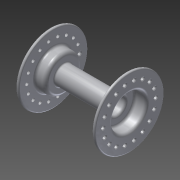
# Autodesk Inventor part: Korpus_piasty
Saved by Autodesk Inventor 2015 (Build 190159000, 159)
## iProperties
Created: 2015-11-24
Part Number: Korpus_piasty
Material: Aluminium AW-7020
Document SubType Name: Modeling
Designer: graaapsik
Density: 2.78 g/cm^3
Appearance: Aluminium AW-7020
Mass: 39.303 g
Surface Area: 181.03 cm^2
Volume: 14.1378 cm^3
Author: graaapsik
Autodesk Inventor part; units mm, degrees
ref_plane "YZ Plane" through (0, 0, 0) normal (1, 0, 0) x (0, 1, 0)
ref_plane "XZ Plane" through (0, 0, 0) normal (0, 1, 0) x (-1, 0, 0)
ref_plane "XY Plane" through (0, 0, 0) normal (0, 0, 1) x (1, 0, 0)
sketch "Szkic1" plane through (0, 0, 0) normal (0, 0, 1) x (1, 0, 0)
  line L0 (-11.9267, 0) -> (11.9804, 0) construction
  line L1 (-21.5, 8) -> (21.5, 8)
  line L2 (0, 16.2765) -> (0, -12.1999) construction
  arc A0 (21.5, 8) -> (22.5, 9) centre (21.5, 9) ccw
  line L3 (22.5, 9) -> (22.5, 12.5)
  arc A1 (25.5, 15.5) -> (22.5, 12.5) centre (25.5, 12.5) ccw
  line L4 (25.5, 15.5) -> (29.25, 15.5)
  arc A2 (29.25, 15.5) -> (31.25, 17.5) centre (29.25, 17.5) ccw
  line L5 (31.25, 17.5) -> (31.25, 28.5)
  arc A3 (32.25, 29.5) -> (31.25, 28.5) centre (32.25, 28.5) ccw
  line L6 (32.25, 29.5) -> (32.75, 29.5)
  line L7 (33.75, 28.5) -> (33.75, 16.98)
  arc A4 (33.75, 28.5) -> (32.75, 29.5) centre (32.75, 28.5) ccw
  line L8 (31.25, 14.48) -> (25.5, 14.48)
  arc A5 (25.5, 14.48) -> (23.52, 12.5) centre (25.5, 12.5) ccw
  line L9 (23.52, 12.5) -> (23.52, 9)
  arc A6 (21.5, 6.98) -> (23.52, 9) centre (21.5, 9) ccw
  line L10 (21.5, 6.98) -> (-21.5, 6.98)
  arc A7 (31.25, 14.48) -> (33.75, 16.98) centre (31.25, 16.98) ccw
  arc A8 (-22.5, 9) -> (-21.5, 8) centre (-21.5, 9) ccw
  line L11 (-22.5, 9) -> (-22.5, 12.5)
  arc A9 (-22.5, 12.5) -> (-25.5, 15.5) centre (-25.5, 12.5) ccw
  line L12 (-25.5, 15.5) -> (-29.25, 15.5)
  arc A10 (-31.25, 17.5) -> (-29.25, 15.5) centre (-29.25, 17.5) ccw
  arc A11 (-33.75, 16.98) -> (-31.25, 14.48) centre (-31.25, 16.98) ccw
  line L13 (-31.25, 14.48) -> (-25.5, 14.48)
  arc A12 (-23.52, 12.5) -> (-25.5, 14.48) centre (-25.5, 12.5) ccw
  line L14 (-23.52, 12.5) -> (-23.52, 9)
  arc A13 (-23.52, 9) -> (-21.5, 6.98) centre (-21.5, 9) ccw
  line L15 (-31.25, 17.5) -> (-31.25, 28.5)
  arc A14 (-31.25, 28.5) -> (-32.25, 29.5) centre (-32.25, 28.5) ccw
  line L16 (-32.25, 29.5) -> (-32.75, 29.5)
  arc A15 (-32.75, 29.5) -> (-33.75, 28.5) centre (-32.75, 28.5) ccw
  line L17 (-33.75, 28.5) -> (-33.75, 16.98)
  point P0 (0, 0)
  dimension "d1" = 8
  dimension "d8" = 1
  dimension "d16" = 3
  dimension "d18" = 2
  dimension "d20" = 1
  dimension "d22" = 29.5
  dimension "d23" = 1
  dimension "d24" = 2.5
  dimension "d25" = 8.25
  dimension "d27" = 33.75
  dimension "d32" = 1.02
  dimension "d33" = 1.02
  dimension "d34" = 1.02
  dimension "d35" = 1.02
  dimension "d36" = 1.02
  dimension "d38" = 2.5
  dimension "d39" = 15.5
  dimension "d41" = 33.75
  dimension "d42" = 15.5
  dimension "d43" = 1.02
  constraints: 36 end point, 32 point on circle, 32 tangent, 16 centre point, 8 equal radius, 7 equal length, 7 perpendicular, 3 horizontal, 2 point on line, 1 parallel, 1 vertical
  measures "d1" distance between parallel lines of L0 L1
  measures "d8" radius of A0
  measures "d16" radius of A1
  measures "d18" radius of A2
  measures "d20" radius of A3
  measures "d22" distance between parallel lines of L6 L0
  measures "d23" radius of A4
  measures "d24" distance between parallel lines of L7 L5
  measures "d25" distance from line of L7 L4.start
  measures "d27" distance between parallel lines of L7 L2
  measures "d32" distance between parallel lines of L4 L8
  measures "d33" distance between parallel lines of L3 L9
  measures "d34" distance between parallel lines of L1 L10
  measures "d35" radial gap between concentric circles of A0 A6
  measures "d36" radial gap between concentric circles of A1 A5
  measures "d38" radius of A7
  measures "d39" distance between parallel lines of L0 L4
  measures "d41" distance between parallel lines of L2 L17
  measures "d42" distance from line of point (0, 0) L12
  measures "d43" distance between parallel lines of L11 L14
revolve "Piasta" add sketch "Szkic1" angle 360 about axis through (-11.9267, 0, 0) along (1, 0, 0)
sketch "Szkic2" plane through (33.75, 0, 0) normal (1, 0, 0) x (0, 0, -1)
  circle A0 centre (0, 0) radius 28.5 projected
  point P0 (0, 22.5)
  dimension "d44" = 22.5
  constraints: 1 vertical alignment
  measures "d44" distance of A0.centre point (0, 22.5)
hole "Otwór na szprychę" at (33.75, 22.5, 0) direction (-1, 0, 0) diameter 2.8 end through all
chamfer "Faza1" distance 0.5 angle 45 2 edges at (31.25, 22.5, 1.4) (33.75, 22.5, 1.4) measured on face at (32.9167, 22.6127, -1.3955)
chamfer "Faza2" distance 0.5 angle 45 2 edges at (-33.75, 22.5, 1.4) (-31.25, 22.5, 1.4) measured on face at (-32.0833, 22.7246, -1.3819)
pattern_circular "Szyk otworów na szprychy" count 18 over 360 about axis through (32.25, 0, 0) along (1, 0, 0) of "Otwór na szprychę", "Faza1"
